Autodesk Inventor part; units mm, degrees
(part 2 of 2)
sketch "Sketch6" plane through (0, 0, 0) normal (0, -1, 0) x (1, 0, 0)
  line L0 (-44.6545, -40.2355) -> (-44.6545, -44.3733)
  line L1 (-45.4673, -39.4227) -> (-45.4673, -45.1861)
  line L2 (-44.6545, -44.3733) -> (-41.4311, -44.3733)
  line L3 (-41.4311, -44.3733) -> (-41.4311, -40.2355)
  line L4 (-41.4311, -40.2355) -> (-44.6545, -40.2355)
  line L5 (-41.4311, -40.2355) -> (-44.6545, -44.3733) construction
  line L6 (-44.6545, -40.2355) -> (-41.4311, -44.3733) construction
  line L7 (-40.6183, -44.0951) -> (-45.4673, -44.0951)
  line L8 (-40.6183, -40.5137) -> (-45.4673, -44.0951) construction
  line L9 (-45.4673, -40.5137) -> (-40.6183, -40.5137)
  line L10 (-45.4673, -40.5137) -> (-40.6183, -44.0951) construction
  line L11 (-40.6183, -39.4227) -> (-45.4673, -39.4227)
  line L12 (-45.4673, -45.1861) -> (-40.6183, -45.1861)
  line L13 (-45.4673, -39.4227) -> (-40.6183, -45.1861) construction
  line L14 (-40.6183, -39.4227) -> (-45.4673, -45.1861) construction
  line L15 (-40.6183, -45.1861) -> (-40.6183, -39.4227)
  line L16 (-40.6183, -40.5137) -> (-40.6183, -44.0951)
  line L17 (-45.4286, -14.5346) -> (-45.4286, -10.9532)
  line L18 (-45.4673, -44.0951) -> (-45.4673, -40.5137)
  line L19 (-45.671, -53.0938) -> (-45.671, -49.5124)
  line L20 (-44.8582, -53.397) -> (-41.5848, -53.397)
  line L21 (-44.8582, -49.2092) -> (-44.8582, -53.397)
  line L22 (-40.772, -53.0938) -> (-45.671, -53.0938)
  line L23 (-45.671, -54.2098) -> (-40.772, -54.2098)
  line L24 (-41.5848, -49.2092) -> (-44.8582, -49.2092)
  line L25 (-45.671, -48.3964) -> (-45.671, -54.2098)
  line L26 (-44.8582, -49.2092) -> (-41.5848, -53.397) construction
  line L27 (-41.5848, -53.397) -> (-41.5848, -49.2092)
  line L28 (-41.5848, -49.2092) -> (-44.8582, -53.397) construction
  line L29 (-40.772, -49.5124) -> (-45.671, -53.0938) construction
  line L30 (-45.671, -49.5124) -> (-40.772, -49.5124)
  line L31 (-45.671, -49.5124) -> (-40.772, -53.0938) construction
  line L32 (-40.772, -48.3964) -> (-45.671, -48.3964)
  line L33 (-40.772, -48.3964) -> (-45.671, -54.2098) construction
  line L34 (-45.671, -48.3964) -> (-40.772, -54.2098) construction
  line L35 (-40.772, -49.5124) -> (-40.772, -53.0938)
  line L36 (-40.772, -54.2098) -> (-40.772, -48.3964)
  line L37 (-45.5527, -24.9424) -> (-45.5527, -21.361)
  line L38 (-44.7399, -25.1706) -> (-41.6165, -25.1706)
  line L39 (-44.7399, -21.1328) -> (-44.7399, -25.1706)
  line L40 (-40.8037, -24.9424) -> (-45.5527, -24.9424)
  line L41 (-45.5527, -25.9834) -> (-40.8037, -25.9834)
  line L42 (-41.6165, -21.1328) -> (-44.7399, -21.1328)
  line L43 (-41.6165, -25.1706) -> (-41.6165, -21.1328)
  line L44 (-41.6165, -21.1328) -> (-44.7399, -25.1706) construction
  line L45 (-44.7399, -21.1328) -> (-41.6165, -25.1706) construction
  line L46 (-45.5527, -20.32) -> (-45.5527, -25.9834)
  line L47 (-40.8037, -21.361) -> (-45.5527, -24.9424) construction
  line L48 (-45.5527, -21.361) -> (-40.8037, -21.361)
  line L49 (-45.5527, -21.361) -> (-40.8037, -24.9424) construction
  line L50 (-40.8037, -20.32) -> (-45.5527, -20.32)
  line L51 (-45.5527, -20.32) -> (-40.8037, -25.9834) construction
  line L52 (-40.8037, -20.32) -> (-45.5527, -25.9834) construction
  line L53 (-40.8037, -21.361) -> (-40.8037, -24.9424)
  line L54 (-40.8037, -25.9834) -> (-40.8037, -20.32)
  line L55 (-44.6684, -34.9027) -> (-41.495, -34.9027)
  line L56 (-45.4812, -34.6495) -> (-45.4812, -31.0681)
  line L57 (-45.4812, -35.7155) -> (-40.6822, -35.7155)
  line L58 (-40.6822, -34.6495) -> (-45.4812, -34.6495)
  line L59 (-44.6684, -30.8149) -> (-44.6684, -34.9027)
  line L60 (-45.4812, -30.0021) -> (-45.4812, -35.7155)
  line L61 (-41.495, -30.8149) -> (-44.6684, -34.9027) construction
  line L62 (-44.6684, -30.8149) -> (-41.495, -34.9027) construction
  line L63 (-41.495, -34.9027) -> (-41.495, -30.8149)
  line L64 (-40.6822, -31.0681) -> (-40.6822, -34.6495)
  line L65 (-40.6822, -31.0681) -> (-45.4812, -34.6495) construction
  line L66 (-45.4812, -31.0681) -> (-40.6822, -34.6495) construction
  line L67 (-40.6822, -30.0021) -> (-45.4812, -35.7155) construction
  line L68 (-40.6822, -35.7155) -> (-40.6822, -30.0021)
  line L69 (-45.4812, -30.0021) -> (-40.6822, -35.7155) construction
  line L70 (-41.495, -30.8149) -> (-44.6684, -30.8149)
  line L71 (-45.4812, -31.0681) -> (-40.6822, -31.0681)
  line L72 (-40.6822, -30.0021) -> (-45.4812, -30.0021)
  line L73 (-41.5424, -10.75) -> (-44.6158, -10.75)
  line L74 (-44.6158, -10.75) -> (-44.6158, -14.7378)
  line L75 (-45.4286, -10.9532) -> (-40.7296, -10.9532)
  line L76 (-40.7296, -9.9372) -> (-45.4286, -9.9372)
  line L77 (-44.6158, -14.7378) -> (-41.5424, -14.7378)
  line L78 (-41.5424, -10.75) -> (-44.6158, -14.7378) construction
  line L79 (-41.5424, -14.7378) -> (-41.5424, -10.75)
  line L80 (-44.6158, -10.75) -> (-41.5424, -14.7378) construction
  line L81 (-45.4286, -9.9372) -> (-45.4286, -15.5506)
  line L82 (-45.4286, -10.9532) -> (-40.7296, -14.5346) construction
  line L83 (-40.7296, -14.5346) -> (-45.4286, -14.5346)
  line L84 (-45.4286, -15.5506) -> (-40.7296, -15.5506)
  line L85 (-45.4286, -9.9372) -> (-40.7296, -15.5506) construction
  line L86 (-40.7296, -15.5506) -> (-40.7296, -9.9372)
  line L87 (-40.7296, -9.9372) -> (-45.4286, -15.5506) construction
  line L88 (-40.7296, -10.9532) -> (-40.7296, -14.5346)
  line L89 (-40.7296, -10.9532) -> (-45.4286, -14.5346) construction
  point P0 (0, 0)
  point P1 (-43.0428, -42.3044)
  point P2 (-43.0428, -42.3044)
  point P3 (-43.0428, -42.3044)
  point P4 (-43.0428, -42.3044)
  point P5 (-43.0428, -42.3044)
  point P6 (-43.1782, -23.1517)
  point P7 (-43.0791, -12.7439)
  point P8 (-43.0791, -12.7439)
  point P9 (-43.2215, -51.3031)
  point P10 (-43.2215, -51.3031)
  point P11 (-43.2215, -51.3031)
  point P12 (-43.2215, -51.3031)
  point P13 (-43.2215, -51.3031)
  point P14 (-43.0791, -12.7439)
  point P15 (-43.0791, -12.7439)
  point P16 (-43.1782, -23.1517)
  point P17 (-43.1782, -23.1517)
  point P18 (-43.1782, -23.1517)
  point P19 (-43.1782, -23.1517)
  point P20 (-43.0817, -32.8588)
  point P21 (-43.0817, -32.8588)
  point P22 (-43.0817, -32.8588)
  point P23 (-43.0817, -32.8588)
  point P24 (-43.0817, -32.8588)
  point P25 (-43.0791, -12.7439)
  point P26 (-44.8582, -53.0938)
  point P27 (-44.8582, -49.5124)
  point P28 (-44.6545, -40.5137)
  point P29 (-44.6545, -44.0951)
  point P30 (-44.6684, -34.6495)
  point P31 (-44.6684, -31.0681)
  point P32 (-44.7399, -21.361)
  point P33 (-44.7399, -24.9424)
  point P34 (-44.6158, -14.5346)
  point P35 (-44.6158, -10.9532)
  dimension "d150" = 3.9878
  dimension "d151" = 3.0734
  dimension "d152" = 0.8128
  dimension "d153" = 0.8128
  dimension "d154" = 3.5814
  dimension "d155" = 4.0378
  dimension "d156" = 3.1234
  dimension "d157" = 0.8128
  dimension "d158" = 0.8128
  dimension "d159" = 3.5814
  dimension "d160" = 4.0878
  dimension "d161" = 3.1734
  dimension "d162" = 0.8128
  dimension "d163" = 0.8128
  dimension "d164" = 3.5814
  dimension "d165" = 4.1378
  dimension "d166" = 3.2234
  dimension "d167" = 0.8128
  dimension "d168" = 0.8128
  dimension "d169" = 3.5814
  dimension "d170" = 4.1878
  dimension "d171" = 3.2734
  dimension "d172" = 0.8128
  dimension "d173" = 0.8128
  dimension "d174" = 3.5814
  constraints: 180 end point, 50 midpoint, 31 parallel, 15 horizontal, 15 perpendicular, 5 collinear
  measures "d150" distance of L74.start L77.start
  measures "d151" distance between parallel lines of L74 L79
  measures "d152" distance between parallel lines of L84 L77
  measures "d153" distance between parallel lines of L81 L74
  measures "d154" distance between parallel lines of L83 L75
  measures "d155" distance of L39.start L39.end
  measures "d156" distance between parallel lines of L39 L43
  measures "d157" distance between parallel lines of L41 L38
  measures "d158" distance between parallel lines of L46 L39
  measures "d159" distance between parallel lines of L40 L48
  measures "d160" distance of L59.start L55.start
  measures "d161" distance between parallel lines of L59 L63
  measures "d162" distance between parallel lines of L57 L55
  measures "d163" distance between parallel lines of L60 L59
  measures "d164" distance between parallel lines of L58 L71
  measures "d165" distance of L0.start L0.end
  measures "d166" distance between parallel lines of L0 L3
  measures "d167" distance between parallel lines of L12 L2
  measures "d168" distance between parallel lines of L1 L0
  measures "d169" distance between parallel lines of L7 L9
  measures "d170" distance of L24.end L20.start
  measures "d171" distance between parallel lines of L21 L27
  measures "d172" distance between parallel lines of L23 L20
  measures "d173" distance between parallel lines of L25 L21
  measures "d174" distance between parallel lines of L22 L30
extrude "Extrusion7" add sketch "Sketch6" along normal blind 1.524 contours L0 L9 L1 L11 L15 L3 L4 | L0 L2 L3 L7 L15 L12 L1 | L9 L15 L7 L3 | L83 L74 L77 L79 L86 L84 L81 | L81 L76 L86 L75 L79 L73 L74 | L79 L75 L86 L83 | L22 L21 L20 L27 L36 L23 L25 | L25 L32 L36 L30 L27 L24 L21 | L27 L30 L35 L22 | L40 L39 L38 L43 L54 L41 L46 | L46 L50 L54 L48 L43 L42 L39 | L43 L48 L53 L40 | L55 L63 L58 L68 L57 L60 L59 | L63 L71 L64 L58 | L71 L60 L72 L68 L63 L70 L59
body "Solid2"
